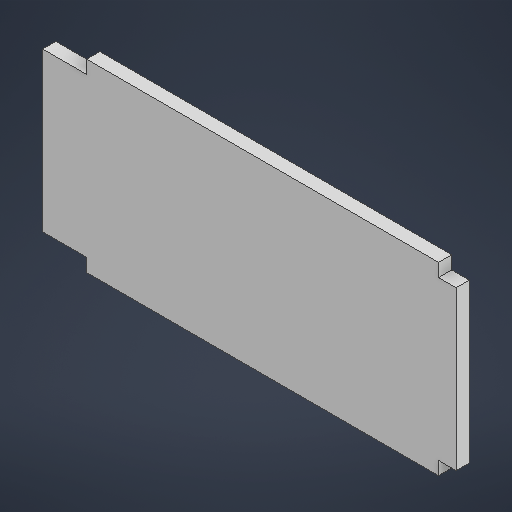
# Autodesk Inventor part: Battary_holder_part2
Saved by Autodesk Inventor 2027 (Build 310192000, 192)
## iProperties
Created: 2026-05-15
Part Number: Battary_holder_part2
Material: Generic
Document SubType Name: Modeling
Designer: alexy
Density: 1 g/cm^3
Appearance: Default
Author: alexy
Autodesk Inventor part; units mm, degrees
ref_plane "YZ Plane" through (0, 0, 0) normal (1, 0, 0) x (0, 1, 0)
ref_plane "XZ Plane" through (0, 0, 0) normal (0, 1, 0) x (-1, 0, 0)
ref_plane "XY Plane" through (0, 0, 0) normal (0, 0, 1) x (1, 0, 0)
sketch "Sketch1" plane through (0, 0, 0) normal (0, 0, 1) x (1, 0, 0)
  line L0 (0, 0) -> (80, 0)
  line L1 (80, 0) -> (80, 42)
  line L2 (80, 42) -> (0, 42)
  line L3 (0, 42) -> (0, 0)
  line L4 (84, 39) -> (80, 39)
  line L5 (80, 39) -> (80, 3)
  line L6 (80, 3) -> (84, 3)
  line L7 (84, 3) -> (84, 39)
  line L8 (84, 39) -> (80, 3) construction
  line L9 (80, 39) -> (84, 3) construction
  line L10 (-10, 39) -> (0, 39)
  line L11 (0, 39) -> (0, 3)
  line L12 (0, 3) -> (-10, 3)
  line L13 (-10, 3) -> (-10, 39)
  line L14 (-10, 39) -> (0, 3) construction
  line L15 (0, 39) -> (-10, 3) construction
  point P0 (82, 21)
  point P1 (-5, 21)
  point P2 (0, 39)
  point P3 (0, 39)
  point P4 (110, 40)
  point P5 (0, 40)
  point P6 (80, 21)
  dimension "d0" = 10
  dimension "d1" = 4
  dimension "d2" = 80
  dimension "d3" = 42
  dimension "d4" = 36
  constraints: 32 end point, 6 parallel, 5 midpoint, 3 horizontal, 3 horizontal alignment, 3 perpendicular, 3 point on line
  measures "d0" distance of L10.start L10.end
  measures "d1" distance of L4.start L4.end
  measures "d2" distance of L0.start L0.end
  measures "d3" distance of L0.end L1.end
  measures "d4" distance of L6.end L4.start
extrude "Extrusion1" add sketch "Sketch1" along normal blind 3
body "Solid1"
